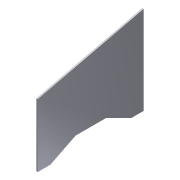
# Autodesk Inventor part: BottomRightSide
Saved by Autodesk Inventor 2014 (Build 180170000, 170)
## iProperties
Created: 2015-01-19
Part Number: BottomRightSide
Material: Generic
Document SubType Name: Modeling
Designer: Peele
Density: 1 g/cm^3
Appearance: White
Author: Peele
Autodesk Inventor part; units mm, degrees
ref_plane "YZ Plane" through (0, 0, 0) normal (1, 0, 0) x (0, 1, 0)
ref_plane "XZ Plane" through (0, 0, 0) normal (0, 1, 0) x (-1, 0, 0)
ref_plane "XY Plane" through (0, 0, 0) normal (0, 0, 1) x (1, 0, 0)
sketch "Sketch1" plane through (0, 0, 0) normal (1, 0, 0) x (0, 1, 0)
  line L0 (-105, -75) -> (105, -75)
  line L1 (105, -75) -> (105, 75)
  line L2 (105, 75) -> (-105, 75)
  line L3 (-105, 75) -> (-105, -75)
  line L4 (-105, -75) -> (105, 75) construction
  line L5 (105, -75) -> (-105, 75) construction
  point P0 (0, 0)
  point P1 (0, 0)
  point P2 (0, 0)
  dimension "d0" = 150
  dimension "d1" = 210
  constraints: 12 end point, 3 midpoint, 2 parallel, 1 coincident, 1 horizontal, 1 perpendicular
  measures "d0" distance of L2.end L0.start
  measures "d1" distance of L1.end L2.end
extrude "Extrusion1" add sketch "Sketch1" along normal blind 3
sketch "Sketch2" plane through (3, 0, 0) normal (1, 0, 0) x (0, 0, -1)
  line L0 (75, -105) -> (75, 105) projected
  line L1 (-75, -105) -> (75, -105) projected
  line L2 (75, 105) -> (100, 105)
  line L3 (100, 105) -> (100, 80)
  line L4 (100, 80) -> (75, 30)
  line L5 (75, 30) -> (75, 105)
  line L6 (75, -105) -> (75, -30)
  line L7 (75, -30) -> (100, -80)
  line L8 (100, -80) -> (100, -105)
  line L9 (100, -105) -> (75, -105)
  point P0 (0, 0)
  dimension "d4" = 25
  dimension "d5" = 50
  constraints: 16 end point, 4 equal length, 2 parallel, 2 perpendicular, 2 point on line, 1 collinear
  measures "d4" distance of L0.end L2.end
  measures "d5" vertical distance of L3.end L4.end
extrude "Extrusion2" add sketch "Sketch2" against normal blind 3
sketch "Sketch3" plane through (3, 0, 0) normal (1, 0, 0) x (0, 0, -1)
  line L0 (-75, 105) -> (-75, -105) projected
  line L1 (-75, -105) -> (100, -105) projected
  line L2 (100, -105) -> (100, -80) projected
  line L3 (-75, 105) -> (-25, -105)
  line L4 (-25, -105) -> (-75, -105)
  line L5 (-75, -105) -> (-75, 105)
  point P0 (0, 0)
  dimension "d8" = 50
  constraints: 6 end point, 2 perpendicular, 1 point on line
  measures "d8" distance from line of L0 L3.end
extrude "Extrusion3" cut sketch "Sketch3" against normal blind 3
body "Solid1"
